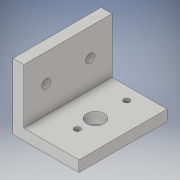
# Autodesk Inventor part: Bumper L-Bracket
Saved by Autodesk Inventor 2019 (Build 230136000, 136)
## iProperties
Created: 2018-11-17
Part Number: Bumper L-Bracket
Material: Generic
Document SubType Name: Modeling
Designer: maste
Density: 1 g/cm^3
Appearance: Default
Author: maste
Autodesk Inventor part; units mm, degrees
ref_plane "YZ Plane" through (0, 0, 0) normal (1, 0, 0) x (0, 1, 0)
ref_plane "XZ Plane" through (0, 0, 0) normal (0, 1, 0) x (-1, 0, 0)
ref_plane "XY Plane" through (0, 0, 0) normal (0, 0, 1) x (1, 0, 0)
sketch "Sketch1" plane through (0, 0, 0) normal (0, 0, 1) x (1, 0, 0)
  line L0 (0, 0) -> (6.35, 0)
  line L1 (6.35, 0) -> (6.35, 38.1)
  line L2 (6.35, 38.1) -> (0, 38.1)
  line L3 (0, 38.1) -> (0, 0)
  line L4 (0, 0) -> (38.1, 0)
  line L5 (38.1, 0) -> (38.1, 6.35)
  line L6 (38.1, 6.35) -> (0, 6.35)
  line L7 (0, 6.35) -> (0, 0)
  dimension "d0" = 6.35
  dimension "d1" = 38.1
  dimension "d2" = 38.1
  dimension "d3" = 6.35
  constraints: 16 end point, 4 parallel, 2 horizontal, 2 perpendicular
  measures "d0" distance of L2.end L1.end
  measures "d1" distance of L1.end L0.end
  measures "d2" distance of L6.end L5.end
  measures "d3" distance of L5.end L4.end
extrude "Extrusion1" add sketch "Sketch1" along normal blind 50.8
sketch "Sketch3" plane through (6.35, 6.35, 0) normal (1, 0, 0) x (0, 0, -1)
  line L0 (0, 0) -> (-50.8, 0) projected
  line L1 (0, 0) -> (0, 15.875)
  line L2 (0, 31.75) -> (0, -6.35) projected
  line L3 (0, 15.875) -> (-50.8, 15.875)
  line L4 (-50.8, 31.75) -> (-50.8, -6.35) projected
  line L5 (-50.8, 15.875) -> (-25.4, 15.875)
  line L6 (-25.4, 15.875) -> (0, 15.875)
  circle A0 centre (-38.1, 15.875) radius 2.54
  circle A1 centre (-12.7, 15.875) radius 2.54
  dimension "d11" = 15.875
  dimension "d12" = 5.08
  dimension "d13" = 5.08
  constraints: 8 end point, 3 midpoint, 2 centre point, 2 perpendicular, 2 point on line
  measures "d11" distance of L0.start L1.end
  measures "d12" diameter of A0
  measures "d13" diameter of A1
extrude "Extrusion3" cut sketch "Sketch3" against normal blind 50.8 contours A1 L3 | L3 A1 | A0 L3 | L3 A0
sketch "Sketch4" plane through (6.35, 6.35, 0) normal (0, 1, 0) x (1, 0, 0)
  line L0 (31.75, 0) -> (0, 0) projected
  line L1 (15.875, 0) -> (15.875, -50.8)
  line L2 (31.75, -50.8) -> (0, -50.8) projected
  line L3 (15.875, 0) -> (15.875, -25.4)
  line L4 (15.875, -25.4) -> (15.875, -50.8)
  circle A0 centre (15.875, -25.4) radius 5.08
  point P0 (-6.35, 0)
  dimension "d16" = 10.16
  constraints: 6 end point, 3 midpoint, 1 centre point, 1 coincident, 1 collinear
  measures "d16" diameter of A0
extrude "Extrusion4" cut sketch "Sketch4" against normal blind 101.6
sketch "Sketch5" plane through (6.35, 6.35, 0) normal (0, 1, 0) x (1, 0, 0)
  circle A0 centre (15.875, -25.4) radius 5.08 projected
  line L0 (15.875, -25.4) -> (15.875, -35.8902)
  circle A1 centre (15.875, -35.8902) radius 1.7018
  line L1 (15.875, -25.4) -> (15.875, -7.3914)
  circle A2 centre (15.875, -7.3914) radius 1.7018
  point P0 (-6.35, 0)
  dimension "d19" = 10.4902
  dimension "d20" = 3.4036
  dimension "d21" = 18.0086
  constraints: 4 end point, 2 centre point, 2 coincident, 2 vertical
  measures "d19" distance of L0.start L0.end
  measures "d20" diameter of A1
  measures "d21" distance of L0.start L1.end
extrude "Extrusion5" cut sketch "Sketch5" against normal blind 50.8 contours A1 | A2
body "Solid1"
